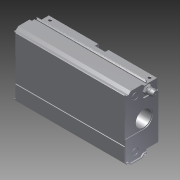
# Autodesk Inventor part: KR45H(A-1)-Slider
Saved by Autodesk Inventor 2011 SP1 (Build 150282100, 282)
## iProperties
Created: 2013-10-24
Part Number: KR45H(A-1)-Slider
Catalog Web Link: www.cadenas.de
Description: LM Guide Actuator - Slider-KR
Vendor: THK
Document SubType Name: Modeling
Designer: PARTuser1
Manufacturer: THK
Density: 1 g/cm^3
Category: PARTsolutions
Company: THK
Title: KR45H(A-1)-Slider
Author: Cadenas PARTsolutions
Comments: KR
PSOL_IDENT_0: {$CADENAS_DATA\23d-libs\thk\lm_guide_actuator\type_kr\parts\lm_g_a_kr_slider.prj},203 {VTYP=3D},{NB=
PSOL_IDENT_1: KR45H(A-1)-Slider},{LINA=KR45H(A-1)-Slider},{NN=LM Guide Actuator - Slider},{DATE=20.05.2010 07:50:2
PSOL_IDENT_2: 6},{GEOMDATE=20.05.2010 07:49:00},{VERSION=},{LINEID=60},{LINESUBID=-1},{WBVAR=TNB,POS}  {NB=KR45H(A
PSOL_IDENT_3: -1)-Slider},{LINA=KR45H(A-1)-Slider},{KT=DUMMY},{ORDER=KR45H},{XTYPE=6.000},{TNB=A},{L=108},{TNB1='A
PSOL_IDENT_4: ','B','C','D'},{POS=1}
CNS_NT: KR
CNS_NB: KR45H(A-1)-Slider
CNS_NBSYN: $ORDER.($TNB.-$POS.)-Slider
CNS_LINA: KR45H(A-1)-Slider
CNS_ORDER: KR45H
CNS_XTYPE: 6.000
CNS_TNB: A
CNS_L: 108.000
CNS_TNB1: 'A','B','C','D'
CNS_POS: 1
SUPPLIER: THK
ARTICLENO: KR45H(A-1)-Slider
BOMINFO: KR45H(A-1)-Slider
CREATOR: CADENAS GmbH
Autodesk Inventor part; units mm, degrees
sketch "Sketch_1" plane through (0, 0, 0) normal (1, 0, 0) x (0, 1, 0)
  line L0 (1.7616, 31.3584) -> (1.5494, 31.1463)
  line L1 (1.5494, 31.1463) -> (2.6, 30.0957)
  line L2 (2.6, 30.0957) -> (2.6, 30)
  line L3 (2.6, 30) -> (1.8, 29.2)
  line L4 (1.8, 29.2) -> (1.8, 28.5)
  line L5 (1.8, 28.5) -> (-0.92, 28.5)
  line L6 (-0.92, 28.5) -> (-3.05, 30.63)
  line L7 (-3.05, 30.63) -> (-13.95, 30.63)
  line L8 (-13.95, 30.63) -> (-16.08, 28.5)
  line L9 (-16.08, 28.5) -> (-18, 28.5)
  line L10 (-18, 28.5) -> (-18.5, 28)
  line L11 (-18.5, 28) -> (-18.5, 14.43)
  arc A0 (-18, 13.93) -> (-18.5, 14.43) centre (-18.5, 13.93) ccw
  line L12 (-18, 13.93) -> (-18, -13.93)
  arc A1 (-18.5, -14.43) -> (-18, -13.93) centre (-18.5, -13.93) ccw
  line L13 (-18.5, -14.43) -> (-18.5, -28)
  line L14 (-18.5, -28) -> (-18, -28.5)
  line L15 (-18, -28.5) -> (-16.08, -28.5)
  line L16 (-16.08, -28.5) -> (-13.95, -30.63)
  line L17 (-13.95, -30.63) -> (-3.05, -30.63)
  line L18 (-3.05, -30.63) -> (-0.92, -28.5)
  line L19 (-0.92, -28.5) -> (1.8, -28.5)
  line L20 (1.8, -28.5) -> (1.8, -29.2)
  line L21 (1.8, -29.2) -> (2.6, -30)
  line L22 (2.6, -30) -> (2.6, -30.0957)
  line L23 (2.6, -30.0957) -> (1.5494, -31.1463)
  line L24 (1.5494, -31.1463) -> (1.7616, -31.3584)
  line L25 (1.7616, -31.3584) -> (2.9, -30.22)
  line L26 (2.9, -30.22) -> (2.9, -28.5)
  line L27 (2.9, -28.5) -> (2.5, -28.5)
  line L28 (2.5, -28.5) -> (2.5, -26.6)
  line L29 (2.5, -26.6) -> (1.8, -26.6)
  line L30 (1.8, -26.6) -> (1.8, -26.5)
  line L31 (1.8, -26.5) -> (13.7, -26.5)
  line L32 (13.7, -26.5) -> (13.9, -26.3)
  line L33 (13.9, -26.3) -> (13.9, 26.3)
  line L34 (13.9, 26.3) -> (13.7, 26.5)
  line L35 (13.7, 26.5) -> (1.8, 26.5)
  line L36 (1.8, 26.5) -> (1.8, 26.6)
  line L37 (1.8, 26.6) -> (2.5, 26.6)
  line L38 (2.5, 26.6) -> (2.5, 28.5)
  line L39 (2.5, 28.5) -> (2.9, 28.5)
  line L40 (2.9, 28.5) -> (2.9, 30.22)
  line L41 (2.9, 30.22) -> (1.7616, 31.3584)
  circle A2 centre (0, 0) radius 7.5
  constraints: 84 end point, 4 point on circle, 3 centre point
extrude "Extrusion1" add sketch "Sketch_1" along normal mid plane 104.6
sketch "Sketch_2" plane through (52.3, 0, 0) normal (1, 0, 0) x (0, 0, -1)
  line L0 (-30.62, -3.07) -> (-30.62, -13.95)
  line L1 (-30.62, -13.95) -> (-28.49, -16.08)
  line L2 (-28.49, -16.08) -> (-28.49, -18.01)
  line L3 (-28.49, -18.01) -> (-8.5, -18.01)
  line L4 (-8.5, -18.01) -> (-8.5, 0)
  arc A0 (0, 8.5) -> (-8.5, 0) centre (0, 0) ccw
  arc A1 (8.5, 0) -> (0, 8.5) centre (0, 0) ccw
  line L5 (8.5, 0) -> (8.5, -18.01)
  line L6 (8.5, -18.01) -> (28.49, -18.01)
  line L7 (28.49, -18.01) -> (28.49, -16.08)
  line L8 (28.49, -16.08) -> (30.62, -13.95)
  line L9 (30.62, -13.95) -> (30.62, -3.07)
  line L10 (30.62, -3.07) -> (28.49, -0.94)
  line L11 (28.49, -0.94) -> (28.49, 1.69)
  line L12 (28.49, 1.69) -> (25.49, 1.69)
  line L13 (25.49, 1.69) -> (25.49, 13.49)
  line L14 (25.49, 13.49) -> (-25.49, 13.49)
  line L15 (-25.49, 13.49) -> (-25.49, 1.69)
  line L16 (-25.49, 1.69) -> (-28.49, 1.69)
  line L17 (-28.49, 1.69) -> (-28.49, -0.94)
  line L18 (-28.49, -0.94) -> (-30.62, -3.07)
  constraints: 38 end point, 4 point on circle, 2 centre point
extrude "Extrusion2" add sketch "Sketch_2" along normal blind 0.5
sketch "Sketch_3" plane through (52.3, 0, 0) normal (1, 0, 0) x (0, 0, -1)
  line L0 (-30.62, -3.06) -> (-30.62, -13.95)
  line L1 (-30.62, -13.95) -> (-28.49, -16.08)
  line L2 (-28.49, -16.08) -> (-28.49, -18.01)
  line L3 (-28.49, -18.01) -> (-27.65, -18.01)
  line L4 (-27.65, -18.01) -> (-27.65, -15.7321)
  line L5 (-27.65, -15.7321) -> (-29.78, -13.6021)
  line L6 (-29.78, -13.6021) -> (-29.78, -3.4079)
  line L7 (-29.78, -3.4079) -> (-27.65, -1.2779)
  line L8 (-27.65, -1.2779) -> (-27.65, 1.69)
  line L9 (-27.65, 1.69) -> (-28.49, 1.69)
  line L10 (-28.49, 1.69) -> (-28.49, -0.93)
  line L11 (-28.49, -0.93) -> (-30.62, -3.06)
  constraints: 24 end point
extrude "Extrusion3" add sketch "Sketch_3" along normal blind 1.7
sketch "Sketch_4" plane through (52.3, 0, 0) normal (1, 0, 0) x (0, 0, -1)
  line L0 (27.65, -18.01) -> (28.49, -18.01)
  line L1 (28.49, -18.01) -> (28.49, -16.08)
  line L2 (28.49, -16.08) -> (30.62, -13.95)
  line L3 (30.62, -13.95) -> (30.62, -3.06)
  line L4 (30.62, -3.06) -> (28.49, -0.93)
  line L5 (28.49, -0.93) -> (28.49, 1.69)
  line L6 (28.49, 1.69) -> (27.65, 1.69)
  line L7 (27.65, 1.69) -> (27.65, -1.2779)
  line L8 (27.65, -1.2779) -> (29.78, -3.4079)
  line L9 (29.78, -3.4079) -> (29.78, -13.6021)
  line L10 (29.78, -13.6021) -> (27.65, -15.7321)
  line L11 (27.65, -15.7321) -> (27.65, -18.01)
  constraints: 24 end point
extrude "Extrusion4" add sketch "Sketch_4" along normal blind 1.7
sketch "Sketch_5" plane through (-52.3, 0, 0) normal (1, 0, 0) x (0, 0, -1)
  line L0 (-30.62, -3.07) -> (-30.62, -13.95)
  line L1 (-30.62, -13.95) -> (-28.49, -16.08)
  line L2 (-28.49, -16.08) -> (-28.49, -18.01)
  line L3 (-28.49, -18.01) -> (-8.5, -18.01)
  line L4 (-8.5, -18.01) -> (-8.5, 0)
  arc A0 (0, 8.5) -> (-8.5, 0) centre (0, 0) ccw
  arc A1 (8.5, 0) -> (0, 8.5) centre (0, 0) ccw
  line L5 (8.5, 0) -> (8.5, -18.01)
  line L6 (8.5, -18.01) -> (28.49, -18.01)
  line L7 (28.49, -18.01) -> (28.49, -16.08)
  line L8 (28.49, -16.08) -> (30.62, -13.95)
  line L9 (30.62, -13.95) -> (30.62, -3.07)
  line L10 (30.62, -3.07) -> (28.49, -0.94)
  line L11 (28.49, -0.94) -> (28.49, 1.69)
  line L12 (28.49, 1.69) -> (25.49, 1.69)
  line L13 (25.49, 1.69) -> (25.49, 13.49)
  line L14 (25.49, 13.49) -> (-25.49, 13.49)
  line L15 (-25.49, 13.49) -> (-25.49, 1.69)
  line L16 (-25.49, 1.69) -> (-28.49, 1.69)
  line L17 (-28.49, 1.69) -> (-28.49, -0.94)
  line L18 (-28.49, -0.94) -> (-30.62, -3.07)
  constraints: 38 end point, 4 point on circle, 2 centre point
extrude "Extrusion5" add sketch "Sketch_5" against normal blind 0.5
sketch "Sketch_6" plane through (-52.3, 0, 0) normal (1, 0, 0) x (0, 0, -1)
  line L0 (-30.62, -3.06) -> (-30.62, -13.95)
  line L1 (-30.62, -13.95) -> (-28.49, -16.08)
  line L2 (-28.49, -16.08) -> (-28.49, -18.01)
  line L3 (-28.49, -18.01) -> (-27.65, -18.01)
  line L4 (-27.65, -18.01) -> (-27.65, -15.7321)
  line L5 (-27.65, -15.7321) -> (-29.78, -13.6021)
  line L6 (-29.78, -13.6021) -> (-29.78, -3.4079)
  line L7 (-29.78, -3.4079) -> (-27.65, -1.2779)
  line L8 (-27.65, -1.2779) -> (-27.65, 1.69)
  line L9 (-27.65, 1.69) -> (-28.49, 1.69)
  line L10 (-28.49, 1.69) -> (-28.49, -0.93)
  line L11 (-28.49, -0.93) -> (-30.62, -3.06)
  constraints: 24 end point
extrude "Extrusion6" add sketch "Sketch_6" against normal blind 1.7
sketch "Sketch_7" plane through (-52.3, 0, 0) normal (1, 0, 0) x (0, 0, -1)
  line L0 (27.65, -18.01) -> (28.49, -18.01)
  line L1 (28.49, -18.01) -> (28.49, -16.08)
  line L2 (28.49, -16.08) -> (30.62, -13.95)
  line L3 (30.62, -13.95) -> (30.62, -3.06)
  line L4 (30.62, -3.06) -> (28.49, -0.93)
  line L5 (28.49, -0.93) -> (28.49, 1.69)
  line L6 (28.49, 1.69) -> (27.65, 1.69)
  line L7 (27.65, 1.69) -> (27.65, -1.2779)
  line L8 (27.65, -1.2779) -> (29.78, -3.4079)
  line L9 (29.78, -3.4079) -> (29.78, -13.6021)
  line L10 (29.78, -13.6021) -> (27.65, -15.7321)
  line L11 (27.65, -15.7321) -> (27.65, -18.01)
  constraints: 24 end point
extrude "Extrusion7" add sketch "Sketch_7" against normal blind 1.7
sketch "Sketch_8" plane through (0, 0, 0) normal (1, 0, 0) x (0, 1, 0)
  line L0 (13.7, 26.5) -> (13.7, -26.5)
  line L1 (13.7, -26.5) -> (14.5, -25.7)
  line L2 (14.5, -25.7) -> (14.5, -8)
  line L3 (14.5, -8) -> (14, -7.5)
  line L4 (14, -7.5) -> (14, 7.5)
  line L5 (14, 7.5) -> (14.5, 8)
  line L6 (14.5, 8) -> (14.5, 25.7)
  line L7 (14.5, 25.7) -> (13.7, 26.5)
  constraints: 16 end point
extrude "Extrusion8" add sketch "Sketch_8" along normal mid plane 81
sketch "Sketch_9" plane through (0, 10.5, 0) normal (0, 1, 0) x (1, 0, 0)
  line L0 (-5, -29.15) -> (5, -29.15)
  line L1 (5, -29.15) -> (5, -14.15)
  arc A0 (5, -14.15) -> (-5, -14.15) centre (0, -14.15) ccw
  line L2 (-5, -14.15) -> (-5, -29.15)
  constraints: 6 end point, 2 point on circle, 1 centre point
extrude "Extrusion9" cut sketch "Sketch_9" along normal blind 5
sketch "Sketch_10" plane through (0, 10.5, 0) normal (0, 1, 0) x (1, 0, 0)
  line L0 (-5, 29.15) -> (-5, 14.15)
  arc A0 (-5, 14.15) -> (5, 14.15) centre (0, 14.15) ccw
  line L1 (5, 14.15) -> (5, 29.15)
  line L2 (5, 29.15) -> (-5, 29.15)
  constraints: 6 end point, 2 point on circle, 1 centre point
extrude "Extrusion10" cut sketch "Sketch_10" along normal blind 5
sketch "Sketch_11" plane through (0, -8.5, 0) normal (0, 1, 0) x (1, 0, 0)
  line L0 (53, 23) -> (50.5, 23)
  line L1 (50.5, 25.75) -> (53, 25.75)
  line L2 (53, 25.75) -> (53, 26.05)
  line L3 (53, 26.05) -> (50.5, 26.05)
  line L4 (50.5, 26.05) -> (50.5, 25.75)
  constraints: 10 end point
revolve "Revolution1" cut sketch "Sketch_11" angle 360 about axis through (53, -8.5, -23) along (1, 0, 0)
sketch "Sketch_12" plane through (0, -8.5, 0) normal (0, 1, 0) x (1, 0, 0)
  line L0 (53, -23) -> (50.5, -23)
  line L1 (50.5, -20.25) -> (53, -20.25)
  line L2 (53, -20.25) -> (53, -19.95)
  line L3 (53, -19.95) -> (50.5, -19.95)
  line L4 (50.5, -19.95) -> (50.5, -20.25)
  constraints: 10 end point
revolve "Revolution2" cut sketch "Sketch_12" angle 360 about axis through (53, -8.5, 23) along (1, 0, 0)
sketch "Sketch_13" plane through (0, -8.5, 0) normal (0, 1, 0) x (1, 0, 0)
  line L0 (-50.5, 23) -> (-53, 23)
  line L1 (-53, 25.75) -> (-50.5, 25.75)
  line L2 (-50.5, 25.75) -> (-50.5, 26.05)
  line L3 (-50.5, 26.05) -> (-53, 26.05)
  line L4 (-53, 26.05) -> (-53, 25.75)
  constraints: 10 end point
revolve "Revolution3" cut sketch "Sketch_13" angle 360 about axis through (-50.5, -8.5, -23) along (1, 0, 0)
sketch "Sketch_14" plane through (0, -8.5, 0) normal (0, 1, 0) x (1, 0, 0)
  line L0 (-50.5, -23) -> (-53, -23)
  line L1 (-53, -20.25) -> (-50.5, -20.25)
  line L2 (-50.5, -20.25) -> (-50.5, -19.95)
  line L3 (-50.5, -19.95) -> (-53, -19.95)
  line L4 (-53, -19.95) -> (-53, -20.25)
  constraints: 10 end point
revolve "Revolution4" cut sketch "Sketch_14" angle 360 about axis through (-50.5, -8.5, 23) along (1, 0, 0)
sketch "Sketch15" plane through (-40.5, 14.5, -8) normal (0, 1, 0) x (1, 0, 0)
  point P0 (63.5, 13.5)
hole "Drilling 1" at (23, 14.5, -21.5) direction (0, -1, 0) diameter 4.917 depth 10 tip angle 140 countersink diameter 6 countersink angle 90 thread size "M6x1" class "6H" standard "ISO Metric profile"
pattern_linear "Rectangular Pattern1" count 2 spacing 46 along (-1, 0, 0) count 2 spacing 43 along (0, 0, 1) of "Drilling 1"
sketch "Sketch16" plane through (0, 10.5, 0) normal (0, 1, 0) x (1, 0, 0)
  point P0 (0, 23)
hole "Drilling 2" at (0, 10.5, -23) direction (0, -1, 0) diameter 2.459 depth 7 tip angle 140 countersink diameter 3 countersink angle 90 thread size "M3x0.5" class "6H" standard "ISO Metric profile"
sketch "Sketch17" plane through (0, 10.5, 0) normal (0, 1, 0) x (1, 0, 0)
  point P0 (0, -23)
hole "Drilling 3" at (0, 10.5, 23) direction (0, -1, 0) diameter 2.459 depth 7 tip angle 140 countersink diameter 3 countersink angle 90 thread size "M3x0.5" class "6H" standard "ISO Metric profile"
sketch "Sketch18" plane through (-52.3, 1.8, 26.5) normal (0, 0, 1) x (1, 0, 0)
  point P0 (100, 8.6)
hole "Drilling 4" at (47.7, 10.4, 26.5) direction (0, 0, -1) diameter 2.459 depth 4 tip angle 140 countersink diameter 3 countersink angle 90 thread size "M3x0.5" class "6H" standard "ISO Metric profile"
sketch "Sketch19" plane through (-52.3, 1.8, 26.5) normal (0, 0, 1) x (1, 0, 0)
  point P0 (4.6, 8.6)
hole "Drilling 5" at (-47.7, 10.4, 26.5) direction (0, 0, -1) diameter 2.459 depth 4 tip angle 140 countersink diameter 3 countersink angle 90 thread size "M3x0.5" class "6H" standard "ISO Metric profile"
sketch "Sketch20" plane through (52.3, 1.8, -26.5) normal (0, 0, -1) x (-1, 0, 0)
  point P0 (4.6, 8.6)
hole "Drilling 6" at (47.7, 10.4, -26.5) direction (0, 0, 1) diameter 2.459 depth 4 tip angle 140 countersink diameter 3 countersink angle 90 thread size "M3x0.5" class "6H" standard "ISO Metric profile"
sketch "Sketch21" plane through (52.3, 1.8, -26.5) normal (0, 0, -1) x (-1, 0, 0)
  point P0 (100, 8.6)
hole "Drilling 7" at (-47.7, 10.4, -26.5) direction (0, 0, 1) diameter 2.459 depth 4 tip angle 140 countersink diameter 3 countersink angle 90 thread size "M3x0.5" class "6H" standard "ISO Metric profile"
sketch "Sketch_26" plane through (0, 4, 0) normal (0, 1, 0) x (1, 0, 0)
  line L0 (51.5, -22) -> (59.8, -22)
  arc A0 (59.6, -22.8246) -> (59.8, -22) centre (58, -22) ccw
  line L1 (59.6, -22.8246) -> (59.6, -24.4)
  line L2 (59.6, -24.4) -> (56.9, -25.3)
  line L3 (56.9, -25.3) -> (55.5758, -24.8616)
  arc A1 (55.5758, -24.8616) -> (54.7615, -24.9449) centre (55.2615, -25.8109) ccw
  line L4 (54.7615, -24.9449) -> (53.8, -25.5)
  line L5 (53.8, -25.5) -> (53.5452, -26.2)
  line L6 (53.5452, -26.2) -> (51.7548, -26.2)
  line L7 (51.7548, -26.2) -> (51.5, -25.5)
  line L8 (51.5, -25.5) -> (51.5, -22)
  line L9 (51.5, -22) -> (59.8, -22)
  constraints: 20 end point, 4 point on circle, 2 centre point
revolve "Revolution5" add sketch "Sketch_26" angle 360 about axis through (51.5, 4, 22) along (-1, 0, 0)
sketch "Sketch_27" plane through (51.5, 0, 0) normal (1, 0, 0) x (0, 0, -1)
  line L0 (-27.5, -2) -> (-19, -2)
  line L1 (-19, -2) -> (-17, 0)
  line L2 (-17, 0) -> (-17, 15)
  line L3 (-17, 15) -> (-27.5, 15)
  line L4 (-27.5, 15) -> (-27.5, -2)
  line L5 (-25.5, 6.0207) -> (-25.5, 1.9793)
  line L6 (-25.5, 1.9793) -> (-22, -0.0415)
  line L7 (-22, -0.0415) -> (-18.5, 1.9793)
  line L8 (-18.5, 1.9793) -> (-18.5, 6.0207)
  line L9 (-18.5, 6.0207) -> (-22, 8.0415)
  line L10 (-22, 8.0415) -> (-25.5, 6.0207)
  constraints: 22 end point
extrude "Extrusion11" cut sketch "Sketch_27" along normal blind 5.8
ref_plane "slider_body_XY" through (0, 0, 0) normal (1, 0, 0) x (0, 0, -1)
ref_plane "slider_body_YZ" through (0, 0, 0) normal (0, 0, -1) x (0, 1, 0)
ref_plane "slider_body_ZX" through (0, 0, 0) normal (0, 1, 0) x (1, 0, 0)
ref_plane "slider_sensor_dog_XY" through (0, 10.5, 23) normal (0, 1, 0) x (1, 0, 0)
ref_plane "slider_sensor_dog_YZ" through (0, 10.5, 23) normal (1, 0, 0) x (0, 0, -1)
ref_plane "slider_sensor_dog_ZX" through (0, 10.5, 23) normal (0, 0, -1) x (0, 1, 0)
ref_plane "slider_slider_spacer_XY" through (0, 14.5, 0) normal (0, 1, 0) x (1, 0, 0)
ref_plane "slider_slider_spacer_YZ" through (0, 14.5, 0) normal (1, 0, 0) x (0, 0, -1)
ref_plane "slider_slider_spacer_ZX" through (0, 14.5, 0) normal (0, 0, -1) x (0, 1, 0)
body "Solid1"
